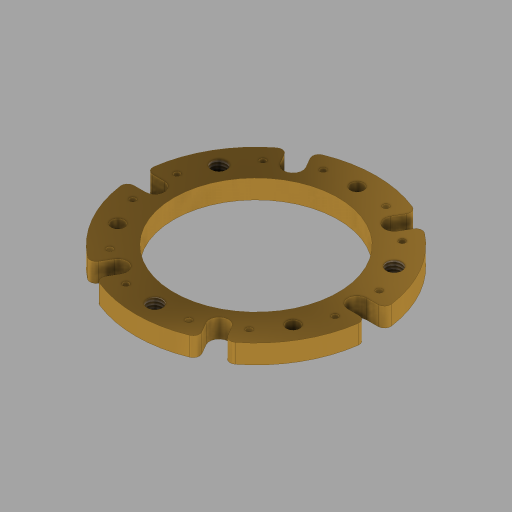
# Autodesk Inventor part: Insert_flange
Saved by Autodesk Inventor 2024 (Build 280153020, 153B)
## iProperties
Created: 2023-09-24
Part Number: Insert_flange
Material: Brass
Document SubType Name: Modeling
Designer: schanen
Density: 8.49 g/cm^3
Appearance: Brass - Polished
Author: schanen
Autodesk Inventor part; units mm, degrees
ref_plane "YZ Plane" through (0, 0, 0) normal (1, 0, 0) x (0, 1, 0)
ref_plane "XZ Plane" through (0, 0, 0) normal (0, 1, 0) x (-1, 0, 0)
ref_plane "XY Plane" through (0, 0, 0) normal (0, 0, 1) x (1, 0, 0)
sketch "Sketch1" plane through (0, 0, 0) normal (0, 0, 1) x (1, 0, 0)
  line L0 (-13, 0) -> (-19, 0)
  line L1 (-19, 0) -> (-19, 3)
  line L2 (-19, 3) -> (-13, 3)
  line L3 (-13, 3) -> (-13, 0)
  line L4 (0, -0.6) -> (0, 3.6) projected
  point P0 (0, 0)
  dimension "d0" = 19
  dimension "d1" = 13
  dimension "d2" = 3
  constraints: 8 end point, 2 parallel, 1 horizontal, 1 perpendicular
  measures "d0" distance from line of point (0, 0) L1
  measures "d1" distance from line of point (0, 0) L3
  measures "d2" distance of L0.end L1.end
revolve "Revolution1" add sketch "Sketch1" angle 360 about axis through (0, -10, 0) along (0, 1, 0)
sketch "Sketch3" plane through (0, 3, 0) normal (0, 1, 0) x (1, 0, 0)
  point P0 (0, 0)
  point P1 (0, 16)
  dimension "d16" = 16
  measures "d16" distance of point (0, 0) point (0, 16)
hole "Hole2" at (0, 3, -16) direction (0, -1, 0) diameter 2.1 end through all
pattern_circular "Circular Pattern1" count 3 over 360 about axis through (0, 1.5, 0) along (0, 1, 0) of "Hole2"
sketch "Sketch4" plane through (0, 3, 0) normal (0, 1, 0) x (1, 0, 0)
  circle A0 centre (-13.8564, -8) radius 1.05 projected
  circle A1 centre (0, 0) radius 16 construction
  circle A2 centre (-16, 0) radius 1.5
  circle A3 centre (0, 0) radius 19 projected
  line L0 (-16, 1.5) -> (-18.9407, 1.5)
  line L1 (-16, -1.5) -> (-18.9407, -1.5)
  arc A4 (-18.9407, 1.5) -> (-18.9407, -1.5) centre (0, 0) ccw
  dimension "d27" = 3
  constraints: 8 point on circle, 4 end point, 3 centre point, 2 coincident, 2 tangent, 1 horizontal, 1 horizontal alignment, 1 parallel
  measures "d27" diameter of A2
extrude "Extrusion1" cut sketch "Sketch4" against normal through all contours A2 | A2 L1 A3 L0 picked at (-18.4455, -0.8441)
fillet "Fillet1" radius 1 2 edges at (-18.9407, 1.5, 1.5) (-18.9407, 1.5, -1.5)
sketch "Sketch5" plane through (-16, 3, 0) normal (0, 1, 0) x (1, 0, 0)
  line L0 (0, -1.5) -> (-1.8255, -1.5) projected
  line L1 (-1.8255, 1.5) -> (0, 1.5) projected
  arc A0 (0, -1.5) -> (0, 1.5) centre (0, 0) ccw projected
  point P0 (16, 0)
  point P1 (0, -3.5)
  point P2 (0, 3.5)
  dimension "d37" = 2
  dimension "d38" = 2
  constraints: 2 vertical alignment
  measures "d37" distance from line of L0 point (0, -3.5)
  measures "d38" distance from line of L1 point (0, 3.5)
hole "Hole3" at (-16, 3, 3.5) at (-16, 3, -3.5) direction (0, -1, 0) diameter 1 end through all
pattern_circular "Circular Pattern4" count 2 over 60 about axis through (0, 1.5, 0) along (0, -1, 0) of "Extrusion1", "Fillet1", "Hole3"
sketch "Sketch6" plane through (-16, 3, 0) normal (0, 1, 0) x (1, 0, 0)
  circle A0 centre (16, 0) radius 16 construction
  arc A1 (0, -1.5) -> (0, 1.5) centre (0, 0) ccw projected
  point P0 (16, 0)
  point P1 (2.1436, 8)
  dimension "d49" = 30
  constraints: 1 coincident, 3 other
hole "Hole4" at (-13.8564, 3, -8) direction (0, -1, 0) diameter 2.459 end through all thread size "M3x0.5" class "6H" standard "ISO Metric profile"
pattern_circular "Circular Pattern5" count 3 over 360 about axis through (0, 1.5, 0) along (0, 1, 0) of "Fillet1", "Extrusion1", "Hole3", "Hole4", "Circular Pattern4"
equation "\"d16\" = CD"
equation "\"d38\" = d37"
equation "\"CD\" = 16"
body "Solid1"
